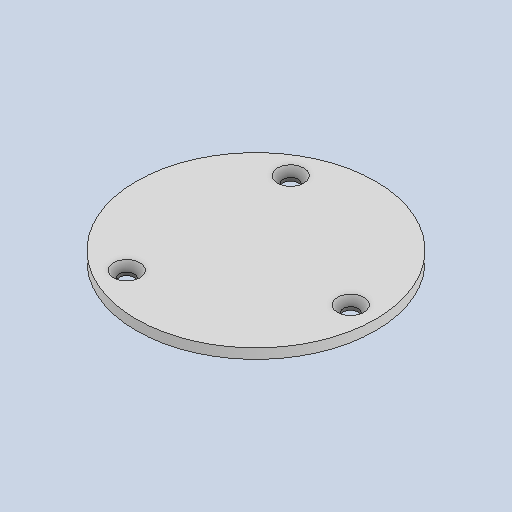
# Autodesk Inventor part: Tapa Soporte rodamientos
Saved by Autodesk Inventor 2023 (Build 270158000, 158)
## iProperties
Created: 2023-04-01
Part Number: Tapa Soporte rodamientos
Material: Genérico
Document SubType Name: Modeling
Designer: sergi
Density: 1 g/cm^3
Appearance: Valor por defecto
Author: sergi
Autodesk Inventor part; units mm, degrees
ref_plane "YZ Plane" through (0, 0, 0) normal (1, 0, 0) x (0, 1, 0)
ref_plane "XZ Plane" through (0, 0, 0) normal (0, 1, 0) x (-1, 0, 0)
ref_plane "XY Plane" through (0, 0, 0) normal (0, 0, 1) x (1, 0, 0)
sketch "Boceto1" plane through (0, 0, 0) normal (0, 1, 0) x (-1, 0, 0)
  circle A0 centre (0, 0) radius 24
  dimension "d0" = 48
  constraints: 1 centre point, 1 coincident
  measures "d0" diameter of A0
extrude "Extrusión1" add sketch "Boceto1" along normal blind 2
sketch "Boceto2" plane through (0, 2, 0) normal (0, 1, 0) x (1, 0, 0)
  circle A0 centre (19.0003, 0.0003) radius 2.2 projected
  circle A1 centre (-9.4997, -16.4542) radius 2.2 projected
  circle A2 centre (-9.4997, 16.4548) radius 2.2 projected
  point P0 (0, 0)
hole "Agujero1" at (-9.4997, 2, 16.4542) at (-9.4997, 2, -16.4548) at (19.0003, 2, -0.0003) direction (0, -1, 0) diameter 3 depth 2 countersink diameter 5.3 countersink angle 80
